Autodesk Fusion 360 part; units mm, degrees
note: some values were not read from the file. Chosen so that the rebuilt part matches the saved one: which bodies a step acts on; which sketch regions a step uses.
(part 2 of 6)
sketch "Sketch12" plane through (0, 0, 0) normal (0, 0, -1) x (1, 0, 0)
  line L0 (173.5975, -110.7442) -> (173.5842, -110.7442)
  line L1 (173.5842, -110.7442) -> (173.5842, -103.6656)
  line L2 (173.5842, -103.6656) -> (173.4543, -103.7337)
  line L3 (173.4543, -103.7337) -> (173.4158, -103.6601)
  line L4 (173.4158, -103.6601) -> (167.5625, -99.9535)
  line L5 (167.5625, -99.9535) -> (158.5133, -104.6955)
  line L6 (158.5133, -104.6955) -> (158.5133, -110.4336)
  line L7 (158.5133, -110.4336) -> (165.6322, -106.703)
  arc A0 (167.2825, -106.8741) -> (165.6322, -106.703) centre (166.3285, -108.0317) ccw
  line L8 (167.2825, -106.8741) -> (167.561, -107.4056)
  line L9 (167.561, -107.4056) -> (167.6652, -107.3509)
  line L10 (167.6652, -107.3509) -> (167.8348, -107.6745)
  arc A1 (167.2024, -109.6993) -> (167.8348, -107.6745) centre (166.5061, -108.3707) ccw
  line L11 (167.2024, -109.6993) -> (148.2048, -119.6546)
  arc A2 (146.4031, -119.3399) -> (148.2048, -119.6546) centre (147.5085, -118.326) ccw
  line L12 (146.4031, -119.3399) -> (146.3131, -119.2418)
  line L13 (146.3131, -119.2418) -> (145.7461, -118.1598)
  arc A3 (146.5446, -116.7055) -> (145.7461, -118.1598) centre (147.2408, -118.0341) ccw
  line L14 (146.5446, -116.7055) -> (157.2133, -111.1148)
  line L15 (157.2133, -111.1148) -> (157.2133, -105.3767)
  line L16 (157.2133, -105.3767) -> (139.9111, -114.4436)
  line L17 (139.9111, -114.4436) -> (139.9111, -121.2175)
  line L18 (139.9111, -121.2175) -> (140.0889, -121.5567)
  line L19 (140.0889, -121.5567) -> (140.0889, -146.1766)
  line L20 (140.0889, -146.1766) -> (146.0889, -149.7175)
  line L21 (146.0889, -149.7175) -> (146.0889, -129.7175)
  arc A4 (147.0889, -128.7175) -> (146.0889, -129.7175) centre (147.0889, -129.7175) ccw
  line L22 (147.0889, -128.7175) -> (148.0889, -128.7175)
  arc A5 (149.0889, -129.7175) -> (148.0889, -128.7175) centre (148.0889, -129.7175) ccw
  line L23 (149.0889, -129.7175) -> (149.0889, -162.7175)
  arc A6 (148.0889, -163.7175) -> (149.0889, -162.7175) centre (148.0889, -162.7175) ccw
  line L24 (148.0889, -163.7175) -> (147.0889, -163.7175)
  arc A7 (146.0889, -162.7175) -> (147.0889, -163.7175) centre (147.0889, -162.7175) ccw
  line L25 (146.0889, -162.7175) -> (146.0563, -152.0206)
  line L26 (146.0563, -152.0206) -> (140.0889, -148.4989)
  line L27 (140.0889, -148.4989) -> (140.0889, -171.2251)
  line L28 (140.0889, -171.2251) -> (164.0889, -171.2251)
  line L29 (164.0889, -171.2251) -> (164.0889, -121.2181)
  line L30 (164.0889, -121.2181) -> (152.0889, -121.2251)
  line L31 (152.0889, -121.2251) -> (173.5975, -110.7442)
  line L32 (164.0889, -121.2181) -> (242.1555, -121.2181)
  line L33 (242.1555, -121.2181) -> (242.1555, -171.2181)
  line L34 (242.1555, -171.2181) -> (164.0889, -171.2181)
  line L35 (164.0889, -171.2181) -> (164.0889, -121.2181)
  dimension "d131" = 50
  constraint horizontal L32
  constraint vertical L33
  constraint horizontal L34
  constraint vertical L35
  constraint coincident L29.end L30.start
  measures "d131" distance of L29.end L34.end
extrude "Extrude19" add sketch "Sketch12" against normal up to surface (2.5 mm away) contours L29 L32 L33 L34 L35 bodies 5 4
sketch "Sketch13" plane through (0, 0, 0) normal (0, 0, -1) x (1, 0, 0)
  line L0 (236.0889, -171.2181) -> (236.0889, -171.2251)
  line L1 (236.0889, -171.2251) -> (260.0889, -171.2251)
  line L2 (260.0889, -171.2251) -> (260.0889, -148.4989)
  line L3 (260.0889, -148.4989) -> (254.1214, -152.0206)
  line L4 (254.1214, -152.0206) -> (254.0889, -162.7175)
  arc A0 (253.0889, -163.7175) -> (254.0889, -162.7175) centre (253.0889, -162.7175) ccw
  line L5 (253.0889, -163.7175) -> (252.0889, -163.7175)
  arc A1 (251.0889, -162.7175) -> (252.0889, -163.7175) centre (252.0889, -162.7175) ccw
  line L6 (251.0889, -162.7175) -> (251.0889, -129.7175)
  arc A2 (252.0889, -128.7175) -> (251.0889, -129.7175) centre (252.0889, -129.7175) ccw
  line L7 (252.0889, -128.7175) -> (253.0889, -128.7175)
  arc A3 (254.0889, -129.7175) -> (253.0889, -128.7175) centre (253.0889, -129.7175) ccw
  line L8 (254.0889, -129.7175) -> (254.0889, -149.7175)
  line L9 (254.0889, -149.7175) -> (260.0889, -146.1766)
  line L10 (260.0889, -146.1766) -> (260.0889, -114.4436)
  line L11 (260.0889, -114.4436) -> (242.9644, -105.4699)
  line L12 (242.9644, -105.4699) -> (242.9644, -111.1148)
  line L13 (242.9644, -111.1148) -> (253.6331, -116.7055)
  arc A4 (254.0423, -119.0481) -> (253.6331, -116.7055) centre (252.9369, -118.0341) ccw
  line L14 (254.0423, -119.0481) -> (253.7746, -119.3399)
  arc A5 (251.973, -119.6546) -> (253.7746, -119.3399) centre (252.6692, -118.326) ccw
  line L15 (251.973, -119.6546) -> (232.9754, -109.6993)
  arc A6 (232.343, -107.6745) -> (232.9754, -109.6993) centre (233.6716, -108.3707) ccw
  line L16 (232.343, -107.6745) -> (232.5206, -107.3354)
  arc A7 (234.5455, -106.703) -> (232.5206, -107.3354) centre (233.8493, -108.0317) ccw
  line L17 (234.5455, -106.703) -> (241.6644, -110.4336)
  line L18 (241.6644, -110.4336) -> (241.6644, -104.7886)
  line L19 (241.6644, -104.7886) -> (232.4375, -99.9535)
  line L20 (232.4375, -99.9535) -> (226.5842, -103.6601)
  line L21 (226.5842, -103.6601) -> (226.5842, -110.7442)
  line L22 (226.5842, -110.7442) -> (248.0889, -121.2175)
  line L23 (248.0889, -121.2175) -> (236.0889, -121.2175)
  line L24 (236.0889, -121.2175) -> (236.0889, -121.2181)
  line L25 (236.0889, -121.2181) -> (164.0889, -121.2181)
  line L26 (164.0889, -121.2181) -> (152.0889, -121.2251)
  line L27 (152.0889, -121.2251) -> (173.5975, -110.7442)
  line L28 (173.5975, -110.7442) -> (173.5842, -110.7442)
  line L29 (173.5842, -110.7442) -> (173.5842, -103.6656)
  line L30 (173.5842, -103.6656) -> (173.4543, -103.7337)
  line L31 (173.4543, -103.7337) -> (173.4158, -103.6601)
  line L32 (173.4158, -103.6601) -> (167.5625, -99.9535)
  line L33 (167.5625, -99.9535) -> (158.5133, -104.6955)
  line L34 (158.5133, -104.6955) -> (158.5133, -110.4336)
  line L35 (158.5133, -110.4336) -> (165.6322, -106.703)
  arc A8 (167.2825, -106.8741) -> (165.6322, -106.703) centre (166.3285, -108.0317) ccw
  line L36 (167.2825, -106.8741) -> (167.561, -107.4056)
  line L37 (167.561, -107.4056) -> (167.6652, -107.3509)
  line L38 (167.6652, -107.3509) -> (167.8348, -107.6745)
  arc A9 (167.2024, -109.6993) -> (167.8348, -107.6745) centre (166.5061, -108.3707) ccw
  line L39 (167.2024, -109.6993) -> (148.2048, -119.6546)
  arc A10 (146.4031, -119.3399) -> (148.2048, -119.6546) centre (147.5085, -118.326) ccw
  line L40 (146.4031, -119.3399) -> (146.3131, -119.2418)
  line L41 (146.3131, -119.2418) -> (145.7461, -118.1598)
  arc A11 (146.5446, -116.7055) -> (145.7461, -118.1598) centre (147.2408, -118.0341) ccw
  line L42 (146.5446, -116.7055) -> (157.2133, -111.1148)
  line L43 (157.2133, -111.1148) -> (157.2133, -105.3767)
  line L44 (157.2133, -105.3767) -> (139.9111, -114.4436)
  line L45 (139.9111, -114.4436) -> (139.9111, -121.2175)
  line L46 (139.9111, -121.2175) -> (140.0889, -121.5567)
  line L47 (140.0889, -121.5567) -> (140.0889, -146.1766)
  line L48 (140.0889, -146.1766) -> (146.0889, -149.7175)
  line L49 (146.0889, -149.7175) -> (146.0889, -129.7175)
  arc A12 (147.0889, -128.7175) -> (146.0889, -129.7175) centre (147.0889, -129.7175) ccw
  line L50 (147.0889, -128.7175) -> (148.0889, -128.7175)
  arc A13 (149.0889, -129.7175) -> (148.0889, -128.7175) centre (148.0889, -129.7175) ccw
  line L51 (149.0889, -129.7175) -> (149.0889, -162.7175)
  arc A14 (148.0889, -163.7175) -> (149.0889, -162.7175) centre (148.0889, -162.7175) ccw
  line L52 (148.0889, -163.7175) -> (147.0889, -163.7175)
  arc A15 (146.0889, -162.7175) -> (147.0889, -163.7175) centre (147.0889, -162.7175) ccw
  line L53 (146.0889, -162.7175) -> (146.0563, -152.0206)
  line L54 (146.0563, -152.0206) -> (140.0889, -148.4989)
  line L55 (140.0889, -148.4989) -> (140.0889, -171.2251)
  line L56 (140.0889, -171.2251) -> (164.0889, -171.2251)
  line L57 (164.0889, -171.2251) -> (164.0889, -171.2181)
  line L58 (164.0889, -171.2181) -> (236.0889, -171.2181)
  line L59 (173.5975, -110.7442) -> (200.0889, -121.2181)
  line L60 (226.5842, -110.7442) -> (200.0889, -121.2181)
  line L61 (152.0889, -171.2251) -> (200.0889, -152.2502)
  line L62 (200.0889, -152.2502) -> (248.0889, -171.2251)
  constraint coincident L27.end L28.start
  constraint midpoint L25 L59.end
  constraint coincident L21.end L22.start
  constraint midpoint L56 L61.start
  constraint parallel L60 L61
  constraint midpoint L1 L62.end
extrude "Extrude20" cut sketch "Sketch13" against normal blind 17 contours L0 L1 L56 L57 L58 L61 L62 bodies 5
extrude "Extrude21" add sketch "Sketch13" against normal up to surface (2.5 mm away) contours L1 L2 L3 L4 A0 L5 A1 L6 A2 L7 A3 L8 L9 L10 L11 L12 L13 A4 L14 A5 L15 A6 L16 A7 L17 L18 L19 L20 L21 L22 L23 L25 L26 L27 L28 L29 L30 L31 L32 L33 L34 L35 A8 L36 L37 L38 A9 L39 A10 L40 L41 A11 L42 L43 L44 L45 L46 L47 L48 L49 A12 L50 A13 L51 A14 L52 A15 L53 L54 L55 L56 L61 L62 | L22 L23 L25 L60 | L25 L26 L27 L59 bodies 5
sketch "holes" plane through (148, 260, 0) normal (0, 0, -1) x (-1, 0, 0)
  line L0 (-38.1657, -108.5347) -> (-40.6657, -108.5347)
  line L1 (-50.7879, -112.8648) -> (-48.2879, -112.8648)
  line L2 (-101.399, -102.868) -> (-102.649, -105.0331)
  line L3 (-10.299, -108.5347) -> (-11.549, -110.6997)
  line L4 (-21.7444, -107.7847) -> (-22.9944, -105.6196)
  line L5 (-15.3722, -109.9497) -> (-12.8722, -109.9497)
  line L6 (-11.6222, -107.7847) -> (-12.8722, -105.6196)
  line L7 (-43.2389, -109.9497) -> (-41.9889, -107.7847)
  line L8 (-5.25, -109.9497) -> (-2.75, -109.9497)
  line L9 (-38.1657, -112.8648) -> (-36.9157, -110.6997)
  line L10 (-7.799, -108.5347) -> (-10.299, -108.5347)
  line L11 (-6.549, -110.6997) -> (-7.799, -108.5347)
  line L12 (-31.8667, -107.7847) -> (-33.1167, -105.6196)
  line L13 (-20.4213, -108.5347) -> (-21.6713, -110.6997)
  line L14 (-33.1167, -109.9497) -> (-31.8667, -107.7847)
  line L15 (-22.9944, -105.6196) -> (-25.4944, -105.6196)
  line L16 (-17.9213, -112.8648) -> (-16.6713, -110.6997)
  line L17 (-15.3722, -105.6196) -> (-16.6222, -107.7847)
  line L18 (-98.899, -102.868) -> (-101.399, -102.868)
  line L19 (-28.0435, -112.8648) -> (-26.7935, -110.6997)
  line L20 (-30.5435, -108.5347) -> (-31.7935, -110.6997)
  line L21 (-26.7935, -110.6997) -> (-28.0435, -108.5347)
  line L22 (-20.4213, -112.8648) -> (-17.9213, -112.8648)
  line L23 (-41.9889, -107.7847) -> (-43.2389, -105.6196)
  line L24 (-28.0435, -108.5347) -> (-30.5435, -108.5347)
  line L25 (-35.6167, -109.9497) -> (-33.1167, -109.9497)
  line L26 (-36.9157, -110.6997) -> (-38.1657, -108.5347)
  line L27 (-40.6657, -108.5347) -> (-41.9157, -110.6997)
  line L28 (-25.4944, -109.9497) -> (-22.9944, -109.9497)
  line L29 (-1.5, -107.7847) -> (-2.75, -105.6196)
  line L30 (-5.25, -105.6196) -> (-6.5, -107.7847)
  line L31 (-21.6713, -110.6997) -> (-20.4213, -112.8648)
  line L32 (-36.8667, -107.7847) -> (-35.6167, -109.9497)
  line L33 (-10.299, -112.8648) -> (-7.799, -112.8648)
  line L34 (-50.7879, -108.5347) -> (-52.0379, -110.6997)
  line L35 (-22.9944, -109.9497) -> (-21.7444, -107.7847)
  line L36 (-102.649, -105.0331) -> (-101.399, -107.1981)
  line L37 (-2.75, -105.6196) -> (-5.25, -105.6196)
  line L38 (-48.2879, -108.5347) -> (-50.7879, -108.5347)
  line L39 (-12.8722, -105.6196) -> (-15.3722, -105.6196)
  line L40 (-40.6657, -112.8648) -> (-38.1657, -112.8648)
  line L41 (-17.9213, -108.5347) -> (-20.4213, -108.5347)
  line L42 (-33.1167, -105.6196) -> (-35.6167, -105.6196)
  line L43 (-41.9157, -110.6997) -> (-40.6657, -112.8648)
  line L44 (-101.399, -107.1981) -> (-98.899, -107.1981)
  line L45 (-16.6713, -110.6997) -> (-17.9213, -108.5347)
  line L46 (-46.9889, -107.7847) -> (-45.7389, -109.9497)
  line L47 (-16.6222, -107.7847) -> (-15.3722, -109.9497)
  line L48 (-7.799, -112.8648) -> (-6.549, -110.6997)
  line L49 (-98.899, -107.1981) -> (-97.649, -105.0331)
  line L50 (-97.649, -105.0331) -> (-98.899, -102.868)
  line L51 (-6.5, -107.7847) -> (-5.25, -109.9497)
  line L52 (-45.7389, -109.9497) -> (-43.2389, -109.9497)
  line L53 (-43.2389, -105.6196) -> (-45.7389, -105.6196)
  line L54 (-11.549, -110.6997) -> (-10.299, -112.8648)
  line L55 (-26.7444, -107.7847) -> (-25.4944, -109.9497)
  line L56 (-82.4778, -107.7847) -> (-83.7278, -105.6196)
  line L57 (-91.2768, -108.5347) -> (-92.5268, -110.6997)
  line L58 (-58.4101, -112.8648) -> (-57.1601, -110.6997)
  line L59 (-96.35, -109.9497) -> (-93.85, -109.9497)
  line L60 (-92.5268, -110.6997) -> (-91.2768, -112.8648)
  line L61 (-48.2879, -112.8648) -> (-47.0379, -110.6997)
  line L62 (-65.9833, -109.9497) -> (-63.4833, -109.9497)
  line L63 (-77.3556, -107.7847) -> (-76.1056, -109.9497)
  line L64 (-73.6056, -105.6196) -> (-76.1056, -105.6196)
  line L65 (-53.3611, -109.9497) -> (-52.1111, -107.7847)
  line L66 (-62.2333, -107.7847) -> (-63.4833, -105.6196)
  line L67 (-98.899, -108.5347) -> (-101.399, -108.5347)
  line L68 (-52.1111, -107.7847) -> (-53.3611, -105.6196)
  line L69 (-91.2768, -112.8648) -> (-88.7768, -112.8648)
  line L70 (-71.0324, -108.5347) -> (-72.2824, -110.6997)
  line L71 (-101.399, -108.5347) -> (-102.649, -110.6997)
  line L72 (-93.85, -105.6196) -> (-96.35, -105.6196)
  line L73 (-86.2278, -105.6196) -> (-87.4778, -107.7847)
  line L74 (-102.649, -110.6997) -> (-101.399, -112.8648)
  line L75 (-101.399, -112.8648) -> (-98.899, -112.8648)
  line L76 (-87.4778, -107.7847) -> (-86.2278, -109.9497)
  line L77 (-88.7768, -112.8648) -> (-87.5268, -110.6997)
  line L78 (-72.3556, -107.7847) -> (-73.6056, -105.6196)
  line L79 (-57.1601, -110.6997) -> (-58.4101, -108.5347)
  line L80 (-58.4101, -108.5347) -> (-60.9101, -108.5347)
  line L81 (-65.9833, -105.6196) -> (-67.2333, -107.7847)
  line L82 (-57.1111, -107.7847) -> (-55.8611, -109.9497)
  line L83 (-86.2278, -109.9497) -> (-83.7278, -109.9497)
  line L84 (-97.6, -107.7847) -> (-96.35, -109.9497)
  line L85 (-68.5324, -108.5347) -> (-71.0324, -108.5347)
  line L86 (-60.9101, -112.8648) -> (-58.4101, -112.8648)
  line L87 (-83.7278, -105.6196) -> (-86.2278, -105.6196)
  line L88 (-67.2824, -110.6997) -> (-68.5324, -108.5347)
  line L89 (-47.0379, -110.6997) -> (-48.2879, -108.5347)
  line L90 (-73.6056, -109.9497) -> (-72.3556, -107.7847)
  line L91 (-97.649, -110.6997) -> (-98.899, -108.5347)
  line L92 (-93.85, -109.9497) -> (-92.6, -107.7847)
  line L93 (-6.5, -113.4513) -> (-5.25, -115.6164)
  line L94 (-5.25, -115.6164) -> (-2.75, -115.6164)
  line L95 (-81.1546, -108.5347) -> (-82.4046, -110.6997)
  line L96 (-98.899, -112.8648) -> (-97.649, -110.6997)
  line L97 (-68.5324, -112.8648) -> (-67.2824, -110.6997)
  line L98 (-60.9101, -108.5347) -> (-62.1601, -110.6997)
  line L99 (-63.4833, -105.6196) -> (-65.9833, -105.6196)
  line L100 (-82.4046, -110.6997) -> (-81.1546, -112.8648)
  line L101 (-77.4046, -110.6997) -> (-78.6546, -108.5347)
  line L102 (-63.4833, -109.9497) -> (-62.2333, -107.7847)
  line L103 (-87.5268, -110.6997) -> (-88.7768, -108.5347)
  line L104 (-92.6, -107.7847) -> (-93.85, -105.6196)
  line L105 (-76.1056, -105.6196) -> (-77.3556, -107.7847)
  line L106 (-71.0324, -112.8648) -> (-68.5324, -112.8648)
  line L107 (-67.2333, -107.7847) -> (-65.9833, -109.9497)
  line L108 (-55.8611, -105.6196) -> (-57.1111, -107.7847)
  line L109 (-88.7768, -108.5347) -> (-91.2768, -108.5347)
  line L110 (-78.6546, -108.5347) -> (-81.1546, -108.5347)
  line L111 (-96.35, -105.6196) -> (-97.6, -107.7847)
  line L112 (-62.1601, -110.6997) -> (-60.9101, -112.8648)
  line L113 (-76.1056, -109.9497) -> (-73.6056, -109.9497)
  line L114 (-72.2824, -110.6997) -> (-71.0324, -112.8648)
  line L115 (-55.8611, -109.9497) -> (-53.3611, -109.9497)
  line L116 (-53.3611, -105.6196) -> (-55.8611, -105.6196)
  line L117 (-45.7389, -105.6196) -> (-46.9889, -107.7847)
  line L118 (-52.0379, -110.6997) -> (-50.7879, -112.8648)
  line L119 (-67.2333, -102.118) -> (-65.9833, -104.2831)
  line L120 (-25.4944, -105.6196) -> (-26.7444, -107.7847)
  line L121 (-30.5435, -112.8648) -> (-28.0435, -112.8648)
  line L122 (-2.75, -109.9497) -> (-1.5, -107.7847)
  line L123 (-12.8722, -109.9497) -> (-11.6222, -107.7847)
  line L124 (-68.5324, -102.868) -> (-71.0324, -102.868)
  line L125 (-31.7935, -110.6997) -> (-30.5435, -112.8648)
  line L126 (-35.6167, -105.6196) -> (-36.8667, -107.7847)
  line L127 (-68.5324, -84.5315) -> (-67.2824, -82.3664)
  line L128 (-71.0324, -90.1981) -> (-68.5324, -90.1981)
  line L129 (-31.7935, -88.0331) -> (-30.5435, -90.1981)
  line L130 (-60.9101, -90.1981) -> (-58.4101, -90.1981)
  line L131 (-41.9889, -85.118) -> (-43.2389, -82.9529)
  line L132 (-48.2879, -90.1981) -> (-47.0379, -88.0331)
  line L133 (-26.7935, -88.0331) -> (-28.0435, -85.868)
  line L134 (-30.5435, -85.868) -> (-31.7935, -88.0331)
  line L135 (-47.0379, -88.0331) -> (-48.2879, -85.868)
  line L136 (-78.6546, -84.5315) -> (-77.4046, -82.3664)
  line L137 (-76.1056, -81.6164) -> (-73.6056, -81.6164)
  line L138 (-35.6167, -87.2831) -> (-33.1167, -87.2831)
  line L139 (-72.2824, -88.0331) -> (-71.0324, -90.1981)
  line L140 (-73.6056, -82.9529) -> (-76.1056, -82.9529)
  line L141 (-76.1056, -82.9529) -> (-77.3556, -85.118)
  line L142 (-55.8611, -87.2831) -> (-53.3611, -87.2831)
  line L143 (-38.1657, -90.1981) -> (-36.9157, -88.0331)
  line L144 (-45.7389, -82.9529) -> (-46.9889, -85.118)
  line L145 (-50.7879, -90.1981) -> (-48.2879, -90.1981)
  line L146 (-57.1601, -88.0331) -> (-58.4101, -85.868)
  line L147 (-62.2333, -85.118) -> (-63.4833, -82.9529)
  line L148 (-36.8667, -85.118) -> (-35.6167, -87.2831)
  line L149 (-28.0435, -90.1981) -> (-26.7935, -88.0331)
  line L150 (-21.7444, -85.118) -> (-22.9944, -82.9529)
  line L151 (-33.1167, -87.2831) -> (-31.8667, -85.118)
  line L152 (-46.9889, -85.118) -> (-45.7389, -87.2831)
  line L153 (-65.9833, -87.2831) -> (-63.4833, -87.2831)
  line L154 (-52.0379, -88.0331) -> (-50.7879, -90.1981)
  line L155 (-67.2824, -88.0331) -> (-68.5324, -85.868)
  line L156 (-50.7879, -85.868) -> (-52.0379, -88.0331)
  line L157 (-41.9157, -88.0331) -> (-40.6657, -90.1981)
  line L158 (-65.9833, -82.9529) -> (-67.2333, -85.118)
  line L159 (-67.2333, -85.118) -> (-65.9833, -87.2831)
  line L160 (-40.6657, -90.1981) -> (-38.1657, -90.1981)
  line L161 (-68.5324, -90.1981) -> (-67.2824, -88.0331)
  line L162 (-36.9157, -88.0331) -> (-38.1657, -85.868)
  line L163 (-43.2389, -87.2831) -> (-41.9889, -85.118)
  line L164 (-22.9944, -87.2831) -> (-21.7444, -85.118)
  line L165 (-63.4833, -87.2831) -> (-62.2333, -85.118)
  line L166 (-28.0435, -85.868) -> (-30.5435, -85.868)
  line L167 (-58.4101, -85.868) -> (-60.9101, -85.868)
  line L168 (-71.0324, -85.868) -> (-72.2824, -88.0331)
  line L169 (-35.6167, -82.9529) -> (-36.8667, -85.118)
  line L170 (-58.4101, -90.1981) -> (-57.1601, -88.0331)
  line L171 (-62.1601, -88.0331) -> (-60.9101, -90.1981)
  line L172 (-76.1056, -87.2831) -> (-73.6056, -87.2831)
  line L173 (-73.6056, -87.2831) -> (-72.3556, -85.118)
  line L174 (-40.6657, -85.868) -> (-41.9157, -88.0331)
  line L175 (-68.5324, -85.868) -> (-71.0324, -85.868)
  line L176 (-77.3556, -85.118) -> (-76.1056, -87.2831)
  line L177 (-55.8611, -82.9529) -> (-57.1111, -85.118)
  line L178 (-31.8667, -85.118) -> (-33.1167, -82.9529)
  line L179 (-52.1111, -85.118) -> (-53.3611, -82.9529)
  line L180 (-72.3556, -85.118) -> (-73.6056, -82.9529)
  line L181 (-33.1167, -82.9529) -> (-35.6167, -82.9529)
  line L182 (-57.1111, -85.118) -> (-55.8611, -87.2831)
  line L183 (-45.7389, -87.2831) -> (-43.2389, -87.2831)
  line L184 (-48.2879, -85.868) -> (-50.7879, -85.868)
  line L185 (-53.3611, -82.9529) -> (-55.8611, -82.9529)
  line L186 (-38.1657, -85.868) -> (-40.6657, -85.868)
  line L187 (-53.3611, -87.2831) -> (-52.1111, -85.118)
  line L188 (-101.399, -85.868) -> (-102.649, -88.0331)
  line L189 (-12.8722, -88.6196) -> (-15.3722, -88.6196)
  line L190 (-98.899, -90.1981) -> (-97.649, -88.0331)
  line L191 (-6.5, -90.7847) -> (-5.25, -92.9497)
  line L192 (-86.2278, -87.2831) -> (-83.7278, -87.2831)
  line L193 (-30.5435, -90.1981) -> (-28.0435, -90.1981)
  line L194 (-11.549, -93.6997) -> (-10.299, -95.8648)
  line L195 (-87.5268, -88.0331) -> (-88.7768, -85.868)
  line L196 (-10.299, -95.8648) -> (-7.799, -95.8648)
  line L197 (-93.85, -82.9529) -> (-96.35, -82.9529)
  line L198 (-102.649, -88.0331) -> (-101.399, -90.1981)
  line L199 (-2.75, -92.9497) -> (-1.5, -90.7847)
  line L200 (-92.5268, -88.0331) -> (-91.2768, -90.1981)
  line L201 (-87.4778, -85.118) -> (-86.2278, -87.2831)
  line L202 (-97.649, -88.0331) -> (-98.899, -85.868)
  line L203 (-77.4046, -88.0331) -> (-78.6546, -85.868)
  line L204 (-96.35, -82.9529) -> (-97.6, -85.118)
  line L205 (-20.4213, -95.8648) -> (-17.9213, -95.8648)
  line L206 (-83.7278, -87.2831) -> (-82.4778, -85.118)
  line L207 (-93.85, -87.2831) -> (-92.6, -85.118)
  line L208 (-7.799, -95.8648) -> (-6.549, -93.6997)
  line L209 (-17.9213, -91.5347) -> (-20.4213, -91.5347)
  line L210 (-97.6, -85.118) -> (-96.35, -87.2831)
  line L211 (-82.4046, -88.0331) -> (-81.1546, -90.1981)
  line L212 (-60.9101, -85.868) -> (-62.1601, -88.0331)
  line L213 (-21.6713, -93.6997) -> (-20.4213, -95.8648)
  line L214 (-22.9944, -82.9529) -> (-25.4944, -82.9529)
  line L215 (-15.3722, -92.9497) -> (-12.8722, -92.9497)
  line L216 (-1.5, -90.7847) -> (-2.75, -88.6196)
  line L217 (-16.6713, -93.6997) -> (-17.9213, -91.5347)
  line L218 (-96.35, -87.2831) -> (-93.85, -87.2831)
  line L219 (-6.549, -93.6997) -> (-7.799, -91.5347)
  line L220 (-63.4833, -82.9529) -> (-65.9833, -82.9529)
  line L221 (-25.4944, -82.9529) -> (-26.7444, -85.118)
  line L222 (-43.2389, -82.9529) -> (-45.7389, -82.9529)
  line L223 (-16.6222, -90.7847) -> (-15.3722, -92.9497)
  line L224 (-81.1546, -90.1981) -> (-78.6546, -90.1981)
  line L225 (-25.4944, -92.9497) -> (-22.9944, -92.9497)
  line L226 (-26.7444, -90.7847) -> (-25.4944, -92.9497)
  line L227 (-22.9944, -88.6196) -> (-25.4944, -88.6196)
  line L228 (-22.9944, -92.9497) -> (-21.7444, -90.7847)
  line L229 (-5.25, -92.9497) -> (-2.75, -92.9497)
  line L230 (-88.7768, -90.1981) -> (-87.5268, -88.0331)
  line L231 (-28.0435, -91.5347) -> (-30.5435, -91.5347)
  line L232 (-2.75, -88.6196) -> (-5.25, -88.6196)
  line L233 (-25.4944, -88.6196) -> (-26.7444, -90.7847)
  line L234 (-101.399, -90.1981) -> (-98.899, -90.1981)
  line L235 (-12.8722, -92.9497) -> (-11.6222, -90.7847)
  line L236 (-21.7444, -90.7847) -> (-22.9944, -88.6196)
  line L237 (-11.6222, -90.7847) -> (-12.8722, -88.6196)
  line L238 (-91.2768, -85.868) -> (-92.5268, -88.0331)
  line L239 (-82.4778, -85.118) -> (-83.7278, -82.9529)
  line L240 (-88.7768, -85.868) -> (-91.2768, -85.868)
  line L241 (-31.7935, -93.6997) -> (-30.5435, -95.8648)
  line L242 (-7.799, -91.5347) -> (-10.299, -91.5347)
  line L243 (-78.6546, -85.868) -> (-81.1546, -85.868)
  line L244 (-98.899, -85.868) -> (-101.399, -85.868)
  line L245 (-10.299, -91.5347) -> (-11.549, -93.6997)
  line L246 (-15.3722, -88.6196) -> (-16.6222, -90.7847)
  line L247 (-78.6546, -90.1981) -> (-77.4046, -88.0331)
  line L248 (-5.25, -88.6196) -> (-6.5, -90.7847)
  line L249 (-30.5435, -91.5347) -> (-31.7935, -93.6997)
  line L250 (-17.9213, -95.8648) -> (-16.6713, -93.6997)
  line L251 (-20.4213, -91.5347) -> (-21.6713, -93.6997)
  line L252 (-86.2278, -82.9529) -> (-87.4778, -85.118)
  line L253 (-30.5435, -95.8648) -> (-28.0435, -95.8648)
  line L254 (-47.0379, -93.6997) -> (-48.2879, -91.5347)
  line L255 (-67.2824, -93.6997) -> (-68.5324, -91.5347)
  line L256 (-81.1546, -85.868) -> (-82.4046, -88.0331)
  line L257 (-38.1657, -95.8648) -> (-36.9157, -93.6997)
  line L258 (-91.2768, -90.1981) -> (-88.7768, -90.1981)
  line L259 (-73.6056, -92.9497) -> (-72.3556, -90.7847)
  line L260 (-53.3611, -92.9497) -> (-52.1111, -90.7847)
  line L261 (-76.1056, -92.9497) -> (-73.6056, -92.9497)
  line L262 (-78.6546, -91.5347) -> (-81.1546, -91.5347)
  line L263 (-48.2879, -95.8648) -> (-47.0379, -93.6997)
  line L264 (-83.7278, -82.9529) -> (-86.2278, -82.9529)
  line L265 (-46.9889, -90.7847) -> (-45.7389, -92.9497)
  line L266 (-48.2879, -91.5347) -> (-50.7879, -91.5347)
  line L267 (-58.4101, -91.5347) -> (-60.9101, -91.5347)
  line L268 (-72.2824, -93.6997) -> (-71.0324, -95.8648)
  line L269 (-55.8611, -88.6196) -> (-57.1111, -90.7847)
  line L270 (-41.9157, -93.6997) -> (-40.6657, -95.8648)
  line L271 (-71.0324, -91.5347) -> (-72.2824, -93.6997)
  line L272 (-50.7879, -91.5347) -> (-52.0379, -93.6997)
  line L273 (-72.3556, -90.7847) -> (-73.6056, -88.6196)
  line L274 (-43.2389, -92.9497) -> (-41.9889, -90.7847)
  line L275 (-71.0324, -95.8648) -> (-68.5324, -95.8648)
  line L276 (-81.1546, -95.8648) -> (-78.6546, -95.8648)
  line L277 (-45.7389, -92.9497) -> (-43.2389, -92.9497)
  line L278 (-50.7879, -95.8648) -> (-48.2879, -95.8648)
  line L279 (-38.1657, -91.5347) -> (-40.6657, -91.5347)
  line L280 (-33.1167, -88.6196) -> (-35.6167, -88.6196)
  line L281 (-82.4046, -93.6997) -> (-81.1546, -95.8648)
  line L282 (-76.1056, -88.6196) -> (-77.3556, -90.7847)
  line L283 (-26.7935, -93.6997) -> (-28.0435, -91.5347)
  line L284 (-67.2333, -90.7847) -> (-65.9833, -92.9497)
  line L285 (-45.7389, -88.6196) -> (-46.9889, -90.7847)
  line L286 (-68.5324, -95.8648) -> (-67.2824, -93.6997)
  line L287 (-77.4046, -93.6997) -> (-78.6546, -91.5347)
  line L288 (-65.9833, -92.9497) -> (-63.4833, -92.9497)
  line L289 (-77.3556, -90.7847) -> (-76.1056, -92.9497)
  line L290 (-73.6056, -88.6196) -> (-76.1056, -88.6196)
  line L291 (-52.1111, -90.7847) -> (-53.3611, -88.6196)
  line L292 (-60.9101, -91.5347) -> (-62.1601, -93.6997)
  line L293 (-78.6546, -95.8648) -> (-77.4046, -93.6997)
  line L294 (-87.4778, -90.7847) -> (-86.2278, -92.9497)
  line L295 (-86.2278, -92.9497) -> (-83.7278, -92.9497)
  line L296 (-35.6167, -88.6196) -> (-36.8667, -90.7847)
  line L297 (-65.9833, -88.6196) -> (-67.2333, -90.7847)
  line L298 (-81.1546, -91.5347) -> (-82.4046, -93.6997)
  line L299 (-92.6, -85.118) -> (-93.85, -82.9529)
  line L300 (-52.0379, -93.6997) -> (-50.7879, -95.8648)
  line L301 (-62.2333, -90.7847) -> (-63.4833, -88.6196)
  line L302 (-53.3611, -88.6196) -> (-55.8611, -88.6196)
  line L303 (-68.5324, -91.5347) -> (-71.0324, -91.5347)
  line L304 (-36.8667, -90.7847) -> (-35.6167, -92.9497)
  line L305 (-33.1167, -94.2863) -> (-35.6167, -94.2863)
  line L306 (-26.7444, -96.4513) -> (-25.4944, -98.6164)
  line L307 (-98.899, -95.8648) -> (-97.649, -93.6997)
  line L308 (-57.1111, -90.7847) -> (-55.8611, -92.9497)
  line L309 (-62.1601, -93.6997) -> (-60.9101, -95.8648)
  line L310 (-36.9157, -93.6997) -> (-38.1657, -91.5347)
  line L311 (-33.1167, -92.9497) -> (-31.8667, -90.7847)
  line L312 (-31.8667, -90.7847) -> (-33.1167, -88.6196)
  line L313 (-35.6167, -92.9497) -> (-33.1167, -92.9497)
  line L314 (-55.8611, -92.9497) -> (-53.3611, -92.9497)
  line L315 (-28.0435, -95.8648) -> (-26.7935, -93.6997)
  line L316 (-57.1601, -93.6997) -> (-58.4101, -91.5347)
  line L317 (-60.9101, -95.8648) -> (-58.4101, -95.8648)
  line L318 (-63.4833, -88.6196) -> (-65.9833, -88.6196)
  line L319 (-58.4101, -95.8648) -> (-57.1601, -93.6997)
  line L320 (-43.2389, -88.6196) -> (-45.7389, -88.6196)
  line L321 (-63.4833, -92.9497) -> (-62.2333, -90.7847)
  line L322 (-40.6657, -91.5347) -> (-41.9157, -93.6997)
  line L323 (-26.7935, -99.3664) -> (-28.0435, -97.2013)
  line L324 (-40.6657, -95.8648) -> (-38.1657, -95.8648)
  line L325 (-41.9889, -90.7847) -> (-43.2389, -88.6196)
  line L326 (-101.399, -91.5347) -> (-102.649, -93.6997)
  line L327 (-15.3722, -98.6164) -> (-12.8722, -98.6164)
  line L328 (-98.899, -91.5347) -> (-101.399, -91.5347)
  line L329 (-88.7768, -95.8648) -> (-87.5268, -93.6997)
  line L330 (-83.7278, -92.9497) -> (-82.4778, -90.7847)
  line L331 (-20.4213, -97.2013) -> (-21.6713, -99.3664)
  line L332 (-6.5, -96.4513) -> (-5.25, -98.6164)
  line L333 (-7.799, -97.2013) -> (-10.299, -97.2013)
  line L334 (-92.6, -90.7847) -> (-93.85, -88.6196)
  line L335 (-97.649, -93.6997) -> (-98.899, -91.5347)
  line L336 (-7.799, -101.5315) -> (-6.549, -99.3664)
  line L337 (-28.0435, -101.5315) -> (-26.7935, -99.3664)
  line L338 (-33.1167, -98.6164) -> (-31.8667, -96.4513)
  line L339 (-22.9944, -94.2863) -> (-25.4944, -94.2863)
  line L340 (-35.6167, -94.2863) -> (-36.8667, -96.4513)
  line L341 (-36.8667, -96.4513) -> (-35.6167, -98.6164)
  line L342 (-87.5268, -93.6997) -> (-88.7768, -91.5347)
  line L343 (-21.7444, -96.4513) -> (-22.9944, -94.2863)
  line L344 (-2.75, -98.6164) -> (-1.5, -96.4513)
  line L345 (-31.8667, -96.4513) -> (-33.1167, -94.2863)
  line L346 (-91.2768, -91.5347) -> (-92.5268, -93.6997)
  line L347 (-16.6713, -99.3664) -> (-17.9213, -97.2013)
  line L348 (-15.3722, -94.2863) -> (-16.6222, -96.4513)
  line L349 (-22.9944, -98.6164) -> (-21.7444, -96.4513)
  line L350 (-35.6167, -98.6164) -> (-33.1167, -98.6164)
  line L351 (-11.6222, -96.4513) -> (-12.8722, -94.2863)
  line L352 (-82.4778, -90.7847) -> (-83.7278, -88.6196)
  line L353 (-93.85, -92.9497) -> (-92.6, -90.7847)
  line L354 (-10.299, -101.5315) -> (-7.799, -101.5315)
  line L355 (-6.549, -99.3664) -> (-7.799, -97.2013)
  line L356 (-28.0435, -97.2013) -> (-30.5435, -97.2013)
  line L357 (-88.7768, -91.5347) -> (-91.2768, -91.5347)
  line L358 (-101.399, -95.8648) -> (-98.899, -95.8648)
  line L359 (-86.2278, -88.6196) -> (-87.4778, -90.7847)
  line L360 (-17.9213, -97.2013) -> (-20.4213, -97.2013)
  line L361 (-30.5435, -101.5315) -> (-28.0435, -101.5315)
  line L362 (-1.5, -96.4513) -> (-2.75, -94.2863)
  line L363 (-16.6222, -96.4513) -> (-15.3722, -98.6164)
  line L364 (-52.1111, -96.4513) -> (-53.3611, -94.2863)
  line L365 (-57.1601, -99.3664) -> (-58.4101, -97.2013)
  line L366 (-65.9833, -94.2863) -> (-67.2333, -96.4513)
  line L367 (-21.6713, -99.3664) -> (-20.4213, -101.5315)
  line L368 (-48.2879, -97.2013) -> (-50.7879, -97.2013)
  line L369 (-52.0379, -99.3664) -> (-50.7879, -101.5315)
  line L370 (-45.7389, -94.2863) -> (-46.9889, -96.4513)
  line L371 (-10.299, -97.2013) -> (-11.549, -99.3664)
  line L372 (-38.1657, -97.2013) -> (-40.6657, -97.2013)
  line L373 (-67.2333, -96.4513) -> (-65.9833, -98.6164)
  line L374 (-20.4213, -101.5315) -> (-17.9213, -101.5315)
  line L375 (-30.5435, -97.2013) -> (-31.7935, -99.3664)
  line L376 (-102.649, -93.6997) -> (-101.399, -95.8648)
  line L377 (-25.4944, -94.2863) -> (-26.7444, -96.4513)
  line L378 (-45.7389, -98.6164) -> (-43.2389, -98.6164)
  line L379 (-68.5324, -97.2013) -> (-71.0324, -97.2013)
  line L380 (-68.5324, -101.5315) -> (-67.2824, -99.3664)
  line L381 (-55.8611, -98.6164) -> (-53.3611, -98.6164)
  line L382 (-47.0379, -99.3664) -> (-48.2879, -97.2013)
  line L383 (-76.1056, -98.6164) -> (-73.6056, -98.6164)
  line L384 (-58.4101, -97.2013) -> (-60.9101, -97.2013)
  line L385 (-65.9833, -98.6164) -> (-63.4833, -98.6164)
  line L386 (-53.3611, -94.2863) -> (-55.8611, -94.2863)
  line L387 (-40.6657, -101.5315) -> (-38.1657, -101.5315)
  line L388 (-77.3556, -96.4513) -> (-76.1056, -98.6164)
  line L389 (-73.6056, -94.2863) -> (-76.1056, -94.2863)
  line L390 (-12.8722, -98.6164) -> (-11.6222, -96.4513)
  line L391 (-12.8722, -94.2863) -> (-15.3722, -94.2863)
  line L392 (-93.85, -88.6196) -> (-96.35, -88.6196)
  line L393 (-5.25, -94.2863) -> (-6.5, -96.4513)
  line L394 (-96.35, -88.6196) -> (-97.6, -90.7847)
  line L395 (-83.7278, -88.6196) -> (-86.2278, -88.6196)
  line L396 (-17.9213, -101.5315) -> (-16.6713, -99.3664)
  line L397 (-11.549, -99.3664) -> (-10.299, -101.5315)
  line L398 (-25.4944, -98.6164) -> (-22.9944, -98.6164)
  line L399 (-31.7935, -99.3664) -> (-30.5435, -101.5315)
  line L400 (-71.0324, -101.5315) -> (-68.5324, -101.5315)
  line L401 (-81.1546, -97.2013) -> (-82.4046, -99.3664)
  line L402 (-5.25, -98.6164) -> (-2.75, -98.6164)
  line L403 (-78.6546, -97.2013) -> (-81.1546, -97.2013)
  line L404 (-43.2389, -94.2863) -> (-45.7389, -94.2863)
  line L405 (-50.7879, -101.5315) -> (-48.2879, -101.5315)
  line L406 (-92.5268, -93.6997) -> (-91.2768, -95.8648)
  line L407 (-2.75, -94.2863) -> (-5.25, -94.2863)
  line L408 (-97.6, -90.7847) -> (-96.35, -92.9497)
  line L409 (-91.2768, -95.8648) -> (-88.7768, -95.8648)
  line L410 (-96.35, -92.9497) -> (-93.85, -92.9497)
  line L411 (-77.4046, -99.3664) -> (-78.6546, -97.2013)
  line L412 (-36.9157, -99.3664) -> (-38.1657, -97.2013)
  line L413 (-48.2879, -101.5315) -> (-47.0379, -99.3664)
  line L414 (-73.6056, -98.6164) -> (-72.3556, -96.4513)
  line L415 (-76.1056, -94.2863) -> (-77.3556, -96.4513)
  line L416 (-83.7278, -94.2863) -> (-86.2278, -94.2863)
  line L417 (-72.3556, -96.4513) -> (-73.6056, -94.2863)
  line L418 (-82.4778, -96.4513) -> (-83.7278, -94.2863)
  line L419 (-55.8611, -94.2863) -> (-57.1111, -96.4513)
  line L420 (-63.4833, -94.2863) -> (-65.9833, -94.2863)
  line L421 (-50.7879, -97.2013) -> (-52.0379, -99.3664)
  line L422 (-88.7768, -97.2013) -> (-91.2768, -97.2013)
  line L423 (-91.2768, -97.2013) -> (-92.5268, -99.3664)
  line L424 (-92.5268, -99.3664) -> (-91.2768, -101.5315)
  line L425 (-46.9889, -96.4513) -> (-45.7389, -98.6164)
  line L426 (-41.9889, -96.4513) -> (-43.2389, -94.2863)
  line L427 (-72.2824, -99.3664) -> (-71.0324, -101.5315)
  line L428 (-71.0324, -97.2013) -> (-72.2824, -99.3664)
  line L429 (-60.9101, -101.5315) -> (-58.4101, -101.5315)
  line L430 (-58.4101, -101.5315) -> (-57.1601, -99.3664)
  line L431 (-86.2278, -94.2863) -> (-87.4778, -96.4513)
  line L432 (-22.9944, -104.2831) -> (-21.7444, -102.118)
  line L433 (-1.5, -102.118) -> (-2.75, -99.9529)
  line L434 (-81.1546, -101.5315) -> (-78.6546, -101.5315)
  line L435 (-21.6713, -105.0331) -> (-20.4213, -107.1981)
  line L436 (-97.649, -99.3664) -> (-98.899, -97.2013)
  line L437 (-67.2824, -99.3664) -> (-68.5324, -97.2013)
  line L438 (-91.2768, -101.5315) -> (-88.7768, -101.5315)
  line L439 (-82.4046, -99.3664) -> (-81.1546, -101.5315)
  line L440 (-63.4833, -98.6164) -> (-62.2333, -96.4513)
  line L441 (-53.3611, -98.6164) -> (-52.1111, -96.4513)
  line L442 (-87.4778, -96.4513) -> (-86.2278, -98.6164)
  line L443 (-60.9101, -97.2013) -> (-62.1601, -99.3664)
  line L444 (-57.1111, -96.4513) -> (-55.8611, -98.6164)
  line L445 (-43.2389, -98.6164) -> (-41.9889, -96.4513)
  line L446 (-62.2333, -96.4513) -> (-63.4833, -94.2863)
  line L447 (-62.1601, -99.3664) -> (-60.9101, -101.5315)
  line L448 (-86.2278, -98.6164) -> (-83.7278, -98.6164)
  line L449 (-41.9157, -99.3664) -> (-40.6657, -101.5315)
  line L450 (-40.6657, -97.2013) -> (-41.9157, -99.3664)
  line L451 (-38.1657, -101.5315) -> (-36.9157, -99.3664)
  line L452 (-98.899, -97.2013) -> (-101.399, -97.2013)
  line L453 (-17.9213, -102.868) -> (-20.4213, -102.868)
  line L454 (-83.7278, -98.6164) -> (-82.4778, -96.4513)
  line L455 (-78.6546, -101.5315) -> (-77.4046, -99.3664)
  line L456 (-101.399, -101.5315) -> (-98.899, -101.5315)
  line L457 (-7.799, -107.1981) -> (-6.549, -105.0331)
  line L458 (-98.899, -101.5315) -> (-97.649, -99.3664)
  line L459 (-16.6713, -105.0331) -> (-17.9213, -102.868)
  line L460 (-93.85, -94.2863) -> (-96.35, -94.2863)
  line L461 (-31.7935, -105.0331) -> (-30.5435, -107.1981)
  line L462 (-25.4944, -99.9529) -> (-26.7444, -102.118)
  line L463 (-10.299, -107.1981) -> (-7.799, -107.1981)
  line L464 (-10.299, -102.868) -> (-11.549, -105.0331)
  line L465 (-38.1657, -107.1981) -> (-36.9157, -105.0331)
  line L466 (-21.7444, -102.118) -> (-22.9944, -99.9529)
  line L467 (-12.8722, -104.2831) -> (-11.6222, -102.118)
  line L468 (-40.6657, -107.1981) -> (-38.1657, -107.1981)
  line L469 (-36.9157, -105.0331) -> (-38.1657, -102.868)
  line L470 (-40.6657, -102.868) -> (-41.9157, -105.0331)
  line L471 (-96.35, -98.6164) -> (-93.85, -98.6164)
  line L472 (-20.4213, -102.868) -> (-21.6713, -105.0331)
  line L473 (-22.9944, -99.9529) -> (-25.4944, -99.9529)
  line L474 (-28.0435, -107.1981) -> (-26.7935, -105.0331)
  line L475 (-33.1167, -99.9529) -> (-35.6167, -99.9529)
  line L476 (-30.5435, -102.868) -> (-31.7935, -105.0331)
  line L477 (-5.25, -99.9529) -> (-6.5, -102.118)
  line L478 (-28.0435, -102.868) -> (-30.5435, -102.868)
  line L479 (-35.6167, -104.2831) -> (-33.1167, -104.2831)
  line L480 (-7.799, -102.868) -> (-10.299, -102.868)
  line L481 (-11.6222, -102.118) -> (-12.8722, -99.9529)
  line L482 (-26.7444, -102.118) -> (-25.4944, -104.2831)
  line L483 (-45.7389, -104.2831) -> (-43.2389, -104.2831)
  line L484 (-2.75, -99.9529) -> (-5.25, -99.9529)
  line L485 (-88.7768, -101.5315) -> (-87.5268, -99.3664)
  line L486 (-92.6, -96.4513) -> (-93.85, -94.2863)
  line L487 (-33.1167, -104.2831) -> (-31.8667, -102.118)
  line L488 (-16.6222, -102.118) -> (-15.3722, -104.2831)
  line L489 (-20.4213, -107.1981) -> (-17.9213, -107.1981)
  line L490 (-46.9889, -102.118) -> (-45.7389, -104.2831)
  line L491 (-35.6167, -99.9529) -> (-36.8667, -102.118)
  line L492 (-15.3722, -104.2831) -> (-12.8722, -104.2831)
  line L493 (-25.4944, -104.2831) -> (-22.9944, -104.2831)
  line L494 (-31.8667, -102.118) -> (-33.1167, -99.9529)
  line L495 (-2.75, -104.2831) -> (-1.5, -102.118)
  line L496 (-6.5, -102.118) -> (-5.25, -104.2831)
  line L497 (-41.9157, -105.0331) -> (-40.6657, -107.1981)
  line L498 (-11.549, -105.0331) -> (-10.299, -107.1981)
  line L499 (-26.7935, -105.0331) -> (-28.0435, -102.868)
  line L500 (-102.649, -99.3664) -> (-101.399, -101.5315)
  line L501 (-97.6, -96.4513) -> (-96.35, -98.6164)
  line L502 (-5.25, -104.2831) -> (-2.75, -104.2831)
  line L503 (-17.9213, -107.1981) -> (-16.6713, -105.0331)
  line L504 (-38.1657, -102.868) -> (-40.6657, -102.868)
  line L505 (-6.549, -105.0331) -> (-7.799, -102.868)
  line L506 (-30.5435, -107.1981) -> (-28.0435, -107.1981)
  line L507 (-36.8667, -102.118) -> (-35.6167, -104.2831)
  line L508 (-47.0379, -105.0331) -> (-48.2879, -102.868)
  line L509 (-86.2278, -104.2831) -> (-83.7278, -104.2831)
  line L510 (-73.6056, -99.9529) -> (-76.1056, -99.9529)
  line L511 (-48.2879, -107.1981) -> (-47.0379, -105.0331)
  line L512 (-88.7768, -102.868) -> (-91.2768, -102.868)
  line L513 (-12.8722, -99.9529) -> (-15.3722, -99.9529)
  line L514 (-71.0324, -102.868) -> (-72.2824, -105.0331)
  line L515 (-87.4778, -102.118) -> (-86.2278, -104.2831)
  line L516 (-78.6546, -107.1981) -> (-77.4046, -105.0331)
  line L517 (-57.1601, -105.0331) -> (-58.4101, -102.868)
  line L518 (-78.6546, -102.868) -> (-81.1546, -102.868)
  line L519 (-93.85, -98.6164) -> (-92.6, -96.4513)
  line L520 (-82.4046, -105.0331) -> (-81.1546, -107.1981)
  line L521 (-81.1546, -107.1981) -> (-78.6546, -107.1981)
  line L522 (-62.2333, -102.118) -> (-63.4833, -99.9529)
  line L523 (-83.7278, -104.2831) -> (-82.4778, -102.118)
  line L524 (-101.399, -97.2013) -> (-102.649, -99.3664)
  line L525 (-63.4833, -104.2831) -> (-62.2333, -102.118)
  line L526 (-57.1111, -102.118) -> (-55.8611, -104.2831)
  line L527 (-72.2824, -105.0331) -> (-71.0324, -107.1981)
  line L528 (-77.3556, -102.118) -> (-76.1056, -104.2831)
  line L529 (-77.4046, -105.0331) -> (-78.6546, -102.868)
  line L530 (-45.7389, -99.9529) -> (-46.9889, -102.118)
  line L531 (-86.2278, -99.9529) -> (-87.4778, -102.118)
  line L532 (-87.5268, -99.3664) -> (-88.7768, -97.2013)
  line L533 (-96.35, -94.2863) -> (-97.6, -96.4513)
  line L534 (-60.9101, -102.868) -> (-62.1601, -105.0331)
  line L535 (-62.1601, -105.0331) -> (-60.9101, -107.1981)
  line L536 (-81.1546, -102.868) -> (-82.4046, -105.0331)
  line L537 (-48.2879, -102.868) -> (-50.7879, -102.868)
  line L538 (-58.4101, -107.1981) -> (-57.1601, -105.0331)
  line L539 (-55.8611, -104.2831) -> (-53.3611, -104.2831)
  line L540 (-76.1056, -99.9529) -> (-77.3556, -102.118)
  line L541 (-15.3722, -99.9529) -> (-16.6222, -102.118)
  line L542 (-91.2768, -102.868) -> (-92.5268, -105.0331)
  line L543 (-82.4778, -102.118) -> (-83.7278, -99.9529)
  line L544 (-83.7278, -99.9529) -> (-86.2278, -99.9529)
  line L545 (-52.1111, -102.118) -> (-53.3611, -99.9529)
  line L546 (-92.5268, -105.0331) -> (-91.2768, -107.1981)
  line L547 (-76.1056, -104.2831) -> (-73.6056, -104.2831)
  line L548 (-72.3556, -102.118) -> (-73.6056, -99.9529)
  line L549 (-58.4101, -102.868) -> (-60.9101, -102.868)
  line L550 (-97.6, -102.118) -> (-96.35, -104.2831)
  line L551 (-53.3611, -99.9529) -> (-55.8611, -99.9529)
  line L552 (-60.9101, -107.1981) -> (-58.4101, -107.1981)
  line L553 (-68.5324, -107.1981) -> (-67.2824, -105.0331)
  line L554 (-91.2768, -107.1981) -> (-88.7768, -107.1981)
  line L555 (-87.5268, -105.0331) -> (-88.7768, -102.868)
  line L556 (-93.85, -99.9529) -> (-96.35, -99.9529)
  line L557 (-96.35, -99.9529) -> (-97.6, -102.118)
  line L558 (-65.9833, -99.9529) -> (-67.2333, -102.118)
  line L559 (-93.85, -104.2831) -> (-92.6, -102.118)
  line L560 (-50.7879, -107.1981) -> (-48.2879, -107.1981)
  line L561 (-65.9833, -104.2831) -> (-63.4833, -104.2831)
  line L562 (-73.6056, -104.2831) -> (-72.3556, -102.118)
  line L563 (-43.2389, -99.9529) -> (-45.7389, -99.9529)
  line L564 (-63.4833, -99.9529) -> (-65.9833, -99.9529)
  line L565 (-55.8611, -99.9529) -> (-57.1111, -102.118)
  line L566 (-88.7768, -107.1981) -> (-87.5268, -105.0331)
  line L567 (-52.0379, -105.0331) -> (-50.7879, -107.1981)
  line L568 (-92.6, -102.118) -> (-93.85, -99.9529)
  line L569 (-67.2824, -105.0331) -> (-68.5324, -102.868)
  line L570 (-41.9889, -102.118) -> (-43.2389, -99.9529)
  line L571 (-43.2389, -104.2831) -> (-41.9889, -102.118)
  line L572 (-53.3611, -104.2831) -> (-52.1111, -102.118)
  line L573 (-96.35, -104.2831) -> (-93.85, -104.2831)
  line L574 (-50.7879, -102.868) -> (-52.0379, -105.0331)
  line L575 (-71.0324, -107.1981) -> (-68.5324, -107.1981)
  line L576 (-6.5, -5.7847) -> (-5.25, -7.9497)
  line L577 (-65.9833, 2.0471) -> (-67.2333, -0.118)
  line L578 (-72.3556, -0.118) -> (-73.6056, 2.0471)
  line L579 (-81.1546, -0.868) -> (-82.4046, -3.0331)
  line L580 (-67.2333, -0.118) -> (-65.9833, -2.2831)
  line L581 (-92.5268, -3.0331) -> (-91.2768, -5.1981)
  line L582 (-47.0379, -3.0331) -> (-48.2879, -0.868)
  line L583 (-101.399, -5.1981) -> (-98.899, -5.1981)
  line L584 (-57.1111, -0.118) -> (-55.8611, -2.2831)
  line L585 (-97.649, -3.0331) -> (-98.899, -0.868)
  line L586 (-55.8611, -2.2831) -> (-53.3611, -2.2831)
  line L587 (-82.4046, -3.0331) -> (-81.1546, -5.1981)
  line L588 (-58.4101, -5.1981) -> (-57.1601, -3.0331)
  line L589 (-68.5324, -0.868) -> (-71.0324, -0.868)
  line L590 (-73.6056, -2.2831) -> (-72.3556, -0.118)
  line L591 (-83.7278, 2.0471) -> (-86.2278, 2.0471)
  line L592 (-87.5268, -3.0331) -> (-88.7768, -0.868)
  line L593 (-58.4101, -0.868) -> (-60.9101, -0.868)
  line L594 (-63.4833, 2.0471) -> (-65.9833, 2.0471)
  line L595 (-97.6, -0.118) -> (-96.35, -2.2831)
  line L596 (-88.7768, -5.1981) -> (-87.5268, -3.0331)
  line L597 (-87.4778, -0.118) -> (-86.2278, -2.2831)
  line L598 (-53.3611, 2.0471) -> (-55.8611, 2.0471)
  line L599 (-76.1056, 2.0471) -> (-77.3556, -0.118)
  line L600 (-93.85, 2.0471) -> (-96.35, 2.0471)
  line L601 (-82.4778, -0.118) -> (-83.7278, 2.0471)
  line L602 (-52.1111, -0.118) -> (-53.3611, 2.0471)
  line L603 (-98.899, -0.868) -> (-101.399, -0.868)
  line L604 (-60.9101, -5.1981) -> (-58.4101, -5.1981)
  line L605 (-5.25, -7.9497) -> (-2.75, -7.9497)
  line L606 (-78.6546, -5.1981) -> (-77.4046, -3.0331)
  line L607 (-60.9101, -0.868) -> (-62.1601, -3.0331)
  line L608 (-63.4833, -2.2831) -> (-62.2333, -0.118)
  line L609 (-78.6546, -0.868) -> (-81.1546, -0.868)
  line L610 (-91.2768, -5.1981) -> (-88.7768, -5.1981)
  line L611 (-68.5324, -5.1981) -> (-67.2824, -3.0331)
  line L612 (-35.6167, -3.6196) -> (-36.8667, -5.7847)
  line L613 (-16.6713, -8.6997) -> (-17.9213, -6.5347)
  line L614 (-30.5435, -10.8648) -> (-28.0435, -10.8648)
  line L615 (-7.799, -6.5347) -> (-10.299, -6.5347)
  line L616 (-2.75, -3.6196) -> (-5.25, -3.6196)
  line L617 (-10.299, -6.5347) -> (-11.549, -8.6997)
  line L618 (-81.1546, -5.1981) -> (-78.6546, -5.1981)
  line L619 (-77.4046, -3.0331) -> (-78.6546, -0.868)
  line L620 (-76.1056, -2.2831) -> (-73.6056, -2.2831)
  line L621 (-62.1601, -3.0331) -> (-60.9101, -5.1981)
  line L622 (-33.1167, -7.9497) -> (-31.8667, -5.7847)
  line L623 (-88.7768, -0.868) -> (-91.2768, -0.868)
  line L624 (-5.25, -3.6196) -> (-6.5, -5.7847)
  line L625 (-35.6167, -7.9497) -> (-33.1167, -7.9497)
  line L626 (-11.6222, -5.7847) -> (-12.8722, -3.6196)
  line L627 (-36.9157, -8.6997) -> (-38.1657, -6.5347)
  line L628 (-28.0435, -6.5347) -> (-30.5435, -6.5347)
  line L629 (-17.9213, -6.5347) -> (-20.4213, -6.5347)
  line L630 (-30.5435, -6.5347) -> (-31.7935, -8.6997)
  line L631 (-36.8667, -5.7847) -> (-35.6167, -7.9497)
  line L632 (-43.2389, -3.6196) -> (-45.7389, -3.6196)
  line L633 (-25.4944, -7.9497) -> (-22.9944, -7.9497)
  line L634 (-11.549, -8.6997) -> (-10.299, -10.8648)
  line L635 (-16.6222, -5.7847) -> (-15.3722, -7.9497)
  line L636 (-7.799, -10.8648) -> (-6.549, -8.6997)
  line L637 (-40.6657, -10.8648) -> (-38.1657, -10.8648)
  line L638 (-45.7389, -7.9497) -> (-43.2389, -7.9497)
  line L639 (-21.6713, -8.6997) -> (-20.4213, -10.8648)
  line L640 (-10.299, -10.8648) -> (-7.799, -10.8648)
  line L641 (-15.3722, -7.9497) -> (-12.8722, -7.9497)
  line L642 (-41.9157, -8.6997) -> (-40.6657, -10.8648)
  line L643 (-28.0435, -10.8648) -> (-26.7935, -8.6997)
  line L644 (-46.9889, -5.7847) -> (-45.7389, -7.9497)
  line L645 (-40.6657, -6.5347) -> (-41.9157, -8.6997)
  line L646 (-21.7444, -5.7847) -> (-22.9944, -3.6196)
  line L647 (-38.1657, -10.8648) -> (-36.9157, -8.6997)
  line L648 (-22.9944, -3.6196) -> (-25.4944, -3.6196)
  line L649 (-20.4213, -6.5347) -> (-21.6713, -8.6997)
  line L650 (-38.1657, -6.5347) -> (-40.6657, -6.5347)
  line L651 (-33.1167, -3.6196) -> (-35.6167, -3.6196)
  line L652 (-41.9889, -5.7847) -> (-43.2389, -3.6196)
  line L653 (-12.8722, -3.6196) -> (-15.3722, -3.6196)
  line L654 (-31.7935, -8.6997) -> (-30.5435, -10.8648)
  line L655 (-48.2879, -6.5347) -> (-50.7879, -6.5347)
  line L656 (-53.3611, -7.9497) -> (-52.1111, -5.7847)
  line L657 (-50.7879, -10.8648) -> (-48.2879, -10.8648)
  line L658 (-53.3611, -3.6196) -> (-55.8611, -3.6196)
  line L659 (-52.1111, -5.7847) -> (-53.3611, -3.6196)
  line L660 (-12.8722, -7.9497) -> (-11.6222, -5.7847)
  line L661 (-17.9213, -10.8648) -> (-16.6713, -8.6997)
  line L662 (-43.2389, -7.9497) -> (-41.9889, -5.7847)
  line L663 (-47.0379, -8.6997) -> (-48.2879, -6.5347)
  line L664 (-55.8611, -3.6196) -> (-57.1111, -5.7847)
  line L665 (-52.0379, -8.6997) -> (-50.7879, -10.8648)
  line L666 (-26.7444, -5.7847) -> (-25.4944, -7.9497)
  line L667 (-57.1111, -5.7847) -> (-55.8611, -7.9497)
  line L668 (-55.8611, -7.9497) -> (-53.3611, -7.9497)
  line L669 (-31.8667, -5.7847) -> (-33.1167, -3.6196)
  line L670 (-25.4944, -3.6196) -> (-26.7444, -5.7847)
  line L671 (-2.75, -7.9497) -> (-1.5, -5.7847)
  line L672 (-50.7879, -6.5347) -> (-52.0379, -8.6997)
  line L673 (-20.4213, -10.8648) -> (-17.9213, -10.8648)
  line L674 (-22.9944, -7.9497) -> (-21.7444, -5.7847)
  line L675 (-48.2879, -10.8648) -> (-47.0379, -8.6997)
  line L676 (-45.7389, -3.6196) -> (-46.9889, -5.7847)
  line L677 (-6.549, -8.6997) -> (-7.799, -6.5347)
  line L678 (-15.3722, -3.6196) -> (-16.6222, -5.7847)
  line L679 (-1.5, -5.7847) -> (-2.75, -3.6196)
  line L680 (-97.6, -5.7847) -> (-96.35, -7.9497)
  line L681 (-91.2768, -6.5347) -> (-92.5268, -8.6997)
  line L682 (-67.2824, -8.6997) -> (-68.5324, -6.5347)
  line L683 (-72.3556, -5.7847) -> (-73.6056, -3.6196)
  line L684 (-87.4778, -5.7847) -> (-86.2278, -7.9497)
  line L685 (-67.2333, -5.7847) -> (-65.9833, -7.9497)
  line L686 (-82.4778, -5.7847) -> (-83.7278, -3.6196)
  line L687 (-93.85, -3.6196) -> (-96.35, -3.6196)
  line L688 (-65.9833, -7.9497) -> (-63.4833, -7.9497)
  line L689 (-88.7768, -6.5347) -> (-91.2768, -6.5347)
  line L690 (-76.1056, -3.6196) -> (-77.3556, -5.7847)
  line L691 (-77.3556, -5.7847) -> (-76.1056, -7.9497)
  line L692 (-68.5324, -6.5347) -> (-71.0324, -6.5347)
  line L693 (-91.2768, -10.8648) -> (-88.7768, -10.8648)
  line L694 (-96.35, -3.6196) -> (-97.6, -5.7847)
  line L695 (-26.7935, -8.6997) -> (-28.0435, -6.5347)
  line L696 (-88.7768, -10.8648) -> (-87.5268, -8.6997)
  line L697 (-62.1601, -8.6997) -> (-60.9101, -10.8648)
  line L698 (-92.6, -5.7847) -> (-93.85, -3.6196)
  line L699 (-5.25, -13.6164) -> (-2.75, -13.6164)
  line L700 (-87.5268, -8.6997) -> (-88.7768, -6.5347)
  line L701 (-73.6056, -3.6196) -> (-76.1056, -3.6196)
  line L702 (-93.85, -7.9497) -> (-92.6, -5.7847)
  line L703 (-73.6056, -7.9497) -> (-72.3556, -5.7847)
  line L704 (-78.6546, -6.5347) -> (-81.1546, -6.5347)
  line L705 (-63.4833, -3.6196) -> (-65.9833, -3.6196)
  line L706 (-98.899, -6.5347) -> (-101.399, -6.5347)
  line L707 (-98.899, -10.8648) -> (-97.649, -8.6997)
  line L708 (-2.75, -13.6164) -> (-1.5, -11.4513)
  line L709 (-1.5, -11.4513) -> (-2.75, -9.2863)
  line L710 (-58.4101, -10.8648) -> (-57.1601, -8.6997)
  line L711 (-57.1601, -8.6997) -> (-58.4101, -6.5347)
  line L712 (-62.2333, -5.7847) -> (-63.4833, -3.6196)
  line L713 (-101.399, -10.8648) -> (-98.899, -10.8648)
  line L714 (-86.2278, -7.9497) -> (-83.7278, -7.9497)
  line L715 (-78.6546, -10.8648) -> (-77.4046, -8.6997)
  line L716 (-71.0324, -6.5347) -> (-72.2824, -8.6997)
  line L717 (-82.4046, -8.6997) -> (-81.1546, -10.8648)
  line L718 (-102.649, -8.6997) -> (-101.399, -10.8648)
  line L719 (-97.649, -8.6997) -> (-98.899, -6.5347)
  line L720 (-81.1546, -10.8648) -> (-78.6546, -10.8648)
  line L721 (-83.7278, -7.9497) -> (-82.4778, -5.7847)
  line L722 (-96.35, -7.9497) -> (-93.85, -7.9497)